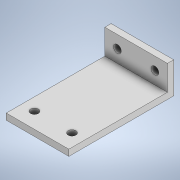
# Autodesk Inventor part: シリンダ固定
Saved by Autodesk Inventor 2021 (Build 250183000, 183)
## iProperties
Created: 2021-10-08
Part Number: シリンダ固定
Material: 一般
Document SubType Name: Modeling
Designer: ryusei
Density: 1 g/cm^3
Appearance: 既定
Author: ryusei
Autodesk Inventor part; units mm, degrees
ref_plane "YZ Plane" through (0, 0, 0) normal (1, 0, 0) x (0, 1, 0)
ref_plane "XZ Plane" through (0, 0, 0) normal (0, 1, 0) x (-1, 0, 0)
ref_plane "XY Plane" through (0, 0, 0) normal (0, 0, 1) x (1, 0, 0)
sketch "スケッチ1" plane through (0, 0, 0) normal (0, 0, 1) x (1, 0, 0)
  line L0 (0, 0) -> (20, 0)
  line L1 (20, 0) -> (20, 10)
  line L2 (20, 10) -> (0, 10)
  line L3 (0, 10) -> (0, 0)
  dimension "d0" = 10
  dimension "d1" = 20
  constraints: 8 end point, 2 parallel, 1 horizontal, 1 perpendicular
  measures "d0" distance between parallel lines of L0 L2
  measures "d1" distance between parallel lines of L1 L3
extrude "押し出し1" add sketch "スケッチ1" along normal blind 2
sketch "スケッチ2" plane through (0, 0, 2) normal (0, 0, 1) x (1, 0, 0)
  line L0 (0, 10) -> (0, 0) projected
  line L1 (20, 0) -> (20, 10) projected
  line L2 (0, 0) -> (20, 0)
  line L3 (20, 0) -> (20, 2)
  line L4 (20, 2) -> (0, 2)
  line L5 (0, 2) -> (0, 0)
  point P0 (0, 2)
  dimension "d4" = 2
  constraints: 8 end point, 2 parallel, 1 horizontal, 1 perpendicular, 1 point on line
  measures "d4" distance between parallel lines of L2 L4
extrude "押し出し2" add sketch "スケッチ2" along normal blind 31.5
sketch "スケッチ3" plane through (0, 0, 2) normal (0, 0, 1) x (1, 0, 0)
  line L0 (20, 2) -> (0, 2) projected
  line L1 (0, 0) -> (20, 0) projected
  line L2 (0, 10) -> (0, 2) projected
  point P0 (16, 6)
  point P1 (4, 6)
  dimension "d8" = 6
  dimension "d9" = 6
  dimension "d10" = 4
  dimension "d11" = 12
  measures "d8" distance from line of L1 point (16, 6)
  measures "d9" distance from line of L1 point (4, 6)
  measures "d10" distance from line of L2 point (4, 6)
  measures "d11" distance of point (16, 6) point (4, 6)
hole "穴1" at (16, 6, 2) at (4, 6, 2) direction (0, 0, -1) diameter 2.5 depth 25 tip angle 118
sketch "スケッチ4" plane through (0, 2, 2) normal (0, 1, 0) x (1, 0, 0)
  line L0 (20, -31.5) -> (0, -31.5) projected
  line L1 (0, 0) -> (0, -31.5) projected
  point P0 (0, 2)
  point P1 (4, -26.5)
  point P2 (16, -26.5)
  dimension "d19" = 5
  dimension "d20" = 5
  dimension "d21" = 12
  dimension "d22" = 4
  measures "d19" distance from line of L0 point (4, -26.5)
  measures "d20" distance from line of L0 point (16, -26.5)
  measures "d21" distance of point (16, -26.5) point (4, -26.5)
  measures "d22" distance from line of L1 point (4, -26.5)
hole "穴2" at (4, 2, 28.5) at (16, 2, 28.5) direction (0, -1, 0) diameter 2.5 depth 25 tip angle 118
